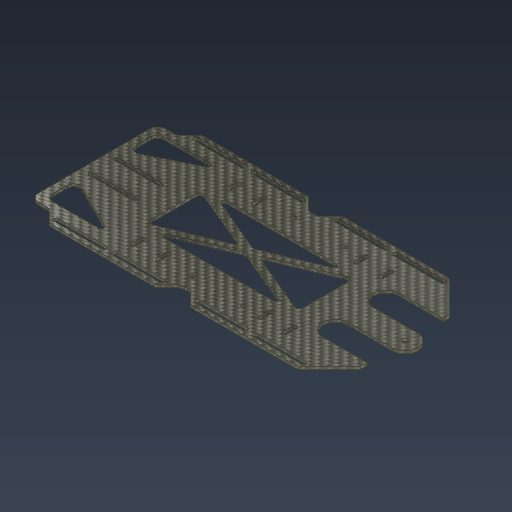
# Autodesk Inventor part: Battery_Tray
Saved by Autodesk Inventor 2024.1 (Build 281209000, 209)
## iProperties
Created: 2023-06-19
Part Number: Battery_Tray
Material: CFRP
Document SubType Name: Modeling
Designer: dzw04
Density: 1.43 g/cm^3
Appearance: Carbon Fiber 1
Mass: 54.159 g
Surface Area: 436.496 cm^2
Volume: 37.8734 cm^3
Author: dzw04
Autodesk Inventor part; units mm, degrees
ref_plane "YZ Plane" through (0, 0, 0) normal (1, 0, 0) x (0, 1, 0)
ref_plane "XZ Plane" through (0, 0, 0) normal (0, 1, 0) x (-1, 0, 0)
ref_plane "XY Plane" through (0, 0, 0) normal (0, 0, 1) x (1, 0, 0)
sketch "Sketch1" plane through (0, 0, 0) normal (0, 1, 0) x (-1, 0, 0)
  line L0 (-110, 36.5) -> (110, 36.5) construction
  line L1 (110, 36.5) -> (110, -36.5) construction
  line L2 (110, -36.5) -> (-110, -36.5) construction
  line L3 (-110, -36.5) -> (-110, 36.5) construction
  line L4 (-110, 36.5) -> (110, -36.5) construction
  line L5 (110, 36.5) -> (-110, -36.5) construction
  line L6 (-110, 29) -> (80, 29) construction
  line L7 (80, 29) -> (80, -29) construction
  line L8 (80, -29) -> (-110, -29) construction
  line L9 (-110, -29) -> (-110, 29) construction
  line L10 (-110, 29) -> (80, -29) construction
  line L11 (80, 29) -> (-110, -29) construction
  line L12 (-110, -29) -> (-110, -34) construction
  line L13 (-110, -34) -> (-60, -34) construction
  line L14 (-60, -34) -> (-50, -34) construction
  line L15 (-50, -34) -> (-70, -34) construction
  line L16 (-50, -34) -> (-50, -41.5) construction
  line L17 (-51.5, -34) -> (-51.5, -41.5)
  line L18 (-48.5, -41.5) -> (-48.5, -34)
  arc A0 (-48.5, -34) -> (-51.5, -34) centre (-50, -34) ccw
  arc A1 (-51.5, -41.5) -> (-48.5, -41.5) centre (-50, -41.5) ccw
  line L19 (-70, -34) -> (-70, -41.5) construction
  line L20 (-71.5, -34) -> (-71.5, -41.5)
  line L21 (-68.5, -41.5) -> (-68.5, -34)
  arc A2 (-68.5, -34) -> (-71.5, -34) centre (-70, -34) ccw
  arc A3 (-71.5, -41.5) -> (-68.5, -41.5) centre (-70, -41.5) ccw
  line L22 (122.5, 50) -> (-122.5, 50)
  line L23 (-122.5, 50) -> (-122.5, -50)
  line L24 (-122.5, -50) -> (122.5, -50)
  line L25 (122.5, -50) -> (122.5, 50)
  line L26 (122.5, 50) -> (-122.5, -50) construction
  line L27 (-122.5, 50) -> (122.5, -50) construction
  line L28 (122.5, 0) -> (-124.7912, 0) construction
  line L29 (-50, -34) -> (30, -34) construction
  line L30 (30, -34) -> (50, -34) construction
  line L31 (30, -34) -> (30, -41.5) construction
  line L32 (28.5, -34) -> (28.5, -41.5)
  line L33 (31.5, -41.5) -> (31.5, -34)
  arc A4 (31.5, -34) -> (28.5, -34) centre (30, -34) ccw
  arc A5 (28.5, -41.5) -> (31.5, -41.5) centre (30, -41.5) ccw
  line L34 (50, -34) -> (50, -41.5) construction
  line L35 (48.5, -34) -> (48.5, -41.5)
  line L36 (51.5, -41.5) -> (51.5, -34)
  arc A6 (51.5, -34) -> (48.5, -34) centre (50, -34) ccw
  arc A7 (48.5, -41.5) -> (51.5, -41.5) centre (50, -41.5) ccw
  line L37 (-110, 0) -> (80, 0) construction
  line L38 (80, 0) -> (80, -10) construction
  line L39 (80, 0) -> (80, 10) construction
  line L40 (80, -10) -> (115, -10) construction
  line L41 (80, -11.5) -> (115, -11.5)
  line L42 (115, -8.5) -> (80, -8.5)
  arc A8 (80, -8.5) -> (80, -11.5) centre (80, -10) ccw
  arc A9 (115, -11.5) -> (115, -8.5) centre (115, -10) ccw
  line L43 (80, 10) -> (115, 10) construction
  line L44 (80, 8.5) -> (115, 8.5)
  line L45 (115, 11.5) -> (80, 11.5)
  arc A10 (80, 11.5) -> (80, 8.5) centre (80, 10) ccw
  arc A11 (115, 8.5) -> (115, 11.5) centre (115, 10) ccw
  line L46 (-60, 34) -> (-50, 34) construction
  line L47 (-50, 34) -> (-70, 34) construction
  line L48 (-50, 34) -> (-50, 41.5) construction
  line L49 (-51.5, 34) -> (-51.5, 41.5)
  line L50 (-48.5, 41.5) -> (-48.5, 34)
  arc A12 (-51.5, 34) -> (-48.5, 34) centre (-50, 34) ccw
  arc A13 (-48.5, 41.5) -> (-51.5, 41.5) centre (-50, 41.5) ccw
  line L51 (-70, 34) -> (-70, 41.5) construction
  line L52 (-71.5, 34) -> (-71.5, 41.5)
  line L53 (-68.5, 41.5) -> (-68.5, 34)
  arc A14 (-71.5, 34) -> (-68.5, 34) centre (-70, 34) ccw
  arc A15 (-68.5, 41.5) -> (-71.5, 41.5) centre (-70, 41.5) ccw
  line L54 (-50, 34) -> (30, 34) construction
  line L55 (30, 34) -> (50, 34) construction
  line L56 (30, 34) -> (30, 41.5) construction
  line L57 (28.5, 34) -> (28.5, 41.5)
  line L58 (31.5, 41.5) -> (31.5, 34)
  arc A16 (28.5, 34) -> (31.5, 34) centre (30, 34) ccw
  arc A17 (31.5, 41.5) -> (28.5, 41.5) centre (30, 41.5) ccw
  line L59 (50, 34) -> (50, 41.5) construction
  line L60 (48.5, 34) -> (48.5, 41.5)
  line L61 (51.5, 41.5) -> (51.5, 34)
  arc A18 (48.5, 34) -> (51.5, 34) centre (50, 34) ccw
  arc A19 (51.5, 41.5) -> (48.5, 41.5) centre (50, 41.5) ccw
  circle A20 centre (-122.5, 0) radius 10
  point P0 (0, 0)
  point P1 (-15, 0)
  point P2 (-50, -37.75)
  point P3 (-70, -37.75)
  point P4 (30, -37.75)
  point P5 (50, -37.75)
  point P6 (97.5, -10)
  point P7 (97.5, 10)
  point P8 (-50, 37.75)
  point P9 (-70, 37.75)
  point P10 (30, 37.75)
  point P11 (50, 37.75)
  point P12 (-122.5, -10)
  point P13 (-122.5, 10)
  dimension "d0" = 220
  dimension "d1" = 73
  dimension "d2" = 190
  dimension "d3" = 58
  dimension "d4" = 5
  dimension "d5" = 50
  dimension "d6" = 10
  dimension "d7" = 20
  dimension "d8" = 7.5
  dimension "d9" = 3
  dimension "d10" = 7.5
  dimension "d11" = 3
  dimension "d12" = 245
  dimension "d13" = 100
  dimension "d16" = 80
  dimension "d17" = 20
  dimension "d18" = 7.5
  dimension "d19" = 3
  dimension "d20" = 7.5
  dimension "d21" = 3
  dimension "d22" = 10
  dimension "d23" = 10
  dimension "d24" = 35
  dimension "d25" = 3
  dimension "d26" = 35
  dimension "d27" = 3
  dimension "d52" = 20
  constraints: 144 end point, 40 point on circle, 29 symmetric about line, 24 tangent, 21 centre point, 17 midpoint, 14 parallel, 11 point on line, 8 perpendicular, 3 horizontal, 1 vertical, 8 other
  measures "d0" distance of L1.end L2.end
  measures "d1" distance of L0.end L1.end
  measures "d2" distance of L7.end L8.end
  measures "d3" distance of L6.end L7.end
  measures "d4" distance of L8.end L12.end
  measures "d5" distance of L12.end L13.end
  measures "d6" distance of L13.end L14.end
  measures "d7" distance of L14.end L15.end
  measures "d8" distance of L14.end L16.end
  measures "d9" diameter of A1
  measures "d10" distance of L15.end L19.end
  measures "d11" diameter of A3
  measures "d12" distance of L24.end L23.end
  measures "d13" distance of L23.end L22.end
  measures "d16" distance of L14.end L29.end
  measures "d17" distance of L29.end L30.end
  measures "d18" distance of L29.end L31.end
  measures "d19" diameter of A5
  measures "d20" distance of L30.end L34.end
  measures "d21" diameter of A7
  measures "d22" distance of L37.end L38.end
  measures "d23" distance of L37.end L39.end
  measures "d24" distance of L38.end L40.end
  measures "d25" diameter of A9
  measures "d26" distance of L39.end L43.end
  measures "d27" diameter of A11
  measures "d52" diameter of A20
extrude "Extrusion1" add sketch "Sketch1" along normal blind 2
sketch "Sketch2" plane through (0, 2, 0) normal (0, 1, 0) x (1, 0, 0)
  line L0 (0, 0) -> (55.5, 0) construction
  line L1 (55.5, 0) -> (55.5, -55) construction
  line L2 (55.5, -55) -> (51.5, -55) construction
  line L3 (51.5, -55) -> (14, -55) construction
  line L4 (51.5, -53.25) -> (14, -53.25)
  line L5 (14, -56.75) -> (51.5, -56.75)
  arc A0 (51.5, -56.75) -> (51.5, -53.25) centre (51.5, -55) ccw
  arc A1 (14, -53.25) -> (14, -56.75) centre (14, -55) ccw
  line L6 (14, -55) -> (28.5, -55) construction
  line L7 (28.5, -55) -> (13.5, -55) construction
  line L8 (0, 0) -> (0, -30) construction
  line L9 (55.5, -55) -> (59.5, -55) construction
  line L10 (59.5, -55) -> (97, -55) construction
  line L11 (59.5, -53.25) -> (97, -53.25)
  line L12 (97, -56.75) -> (59.5, -56.75)
  arc A2 (59.5, -53.25) -> (59.5, -56.75) centre (59.5, -55) ccw
  arc A3 (97, -56.75) -> (97, -53.25) centre (97, -55) ccw
  line L13 (97, -55) -> (82.5, -55) construction
  line L14 (82.5, -55) -> (97.5, -55) construction
  line L15 (82.5, -53.25) -> (97.5, -53.25)
  line L16 (97.5, -56.75) -> (82.5, -56.75)
  arc A4 (82.5, -53.25) -> (82.5, -56.75) centre (82.5, -55) ccw
  arc A5 (97.5, -56.75) -> (97.5, -53.25) centre (97.5, -55) ccw
  line L17 (-122.5, -50) -> (122.5, -50) projected
  line L18 (122.5, -50) -> (109.5711, -50)
  line L19 (107.5, -50) -> (107.5, -60) construction
  line L20 (107.5, -60) -> (97.5, -60) construction
  line L21 (98.9645, -58.5355) -> (106.0355, -51.4645)
  line L22 (95.4289, -60) -> (50.5, -60)
  arc A6 (95.4289, -60) -> (98.9645, -58.5355) centre (95.4289, -55) ccw
  arc A7 (109.5711, -50) -> (106.0355, -51.4645) centre (109.5711, -55) ccw
  line L23 (12.0355, -58.5355) -> (4.9645, -51.4645)
  line L24 (15.5711, -60) -> (50.5, -60)
  arc A8 (12.0355, -58.5355) -> (15.5711, -60) centre (15.5711, -55) ccw
  arc A9 (4.9645, -51.4645) -> (1.4289, -50) centre (1.4289, -55) ccw
  line L25 (-55.5, 0) -> (-55.5, -55) construction
  line L26 (-55.5, -55) -> (-51.5, -55) construction
  line L27 (-51.5, -55) -> (-14, -55) construction
  line L28 (-51.5, -53.25) -> (-14, -53.25)
  line L29 (-14, -56.75) -> (-51.5, -56.75)
  arc A10 (-51.5, -53.25) -> (-51.5, -56.75) centre (-51.5, -55) ccw
  arc A11 (-14, -56.75) -> (-14, -53.25) centre (-14, -55) ccw
  line L30 (-14, -55) -> (-28.5, -55) construction
  line L31 (-28.5, -55) -> (-13.5, -55) construction
  line L32 (-28.5, -53.25) -> (-13.5, -53.25)
  line L33 (-13.5, -56.75) -> (-28.5, -56.75)
  arc A12 (-28.5, -53.25) -> (-28.5, -56.75) centre (-28.5, -55) ccw
  arc A13 (-13.5, -56.75) -> (-13.5, -53.25) centre (-13.5, -55) ccw
  line L34 (-97, -56.75) -> (-59.5, -56.75)
  arc A14 (-59.5, -56.75) -> (-59.5, -53.25) centre (-59.5, -55) ccw
  arc A15 (-97, -53.25) -> (-97, -56.75) centre (-97, -55) ccw
  line L35 (-97, -55) -> (-82.5, -55) construction
  arc A16 (-82.5, -56.75) -> (-82.5, -53.25) centre (-82.5, -55) ccw
  line L36 (-97.5, -56.75) -> (-82.5, -56.75)
  arc A17 (-97.5, -53.25) -> (-97.5, -56.75) centre (-97.5, -55) ccw
  line L37 (-82.5, -55) -> (-97.5, -55) construction
  line L38 (-82.5, -53.25) -> (-97.5, -53.25)
  line L39 (-59.5, -55) -> (-97, -55) construction
  line L40 (-59.5, -53.25) -> (-97, -53.25)
  line L41 (-55.5, -55) -> (-59.5, -55) construction
  line L42 (122.5, -50) -> (-122.5, -50)
  line L43 (-122.5, -50) -> (-109.5711, -50)
  line L44 (-107.5, -50) -> (-107.5, -60) construction
  line L45 (-107.5, -60) -> (-97.5, -60) construction
  line L46 (-98.9645, -58.5355) -> (-106.0355, -51.4645)
  line L47 (-95.4289, -60) -> (-50.5, -60)
  arc A18 (-98.9645, -58.5355) -> (-95.4289, -60) centre (-95.4289, -55) ccw
  arc A19 (-106.0355, -51.4645) -> (-109.5711, -50) centre (-109.5711, -55) ccw
  line L48 (-15.5711, -60) -> (-50.5, -60)
  arc A20 (-15.5711, -60) -> (-12.0355, -58.5355) centre (-15.5711, -55) ccw
  line L49 (-12.0355, -58.5355) -> (-4.9645, -51.4645)
  arc A21 (-1.4289, -50) -> (-4.9645, -51.4645) centre (-1.4289, -55) ccw
  line L50 (55.5, 0) -> (55.5, 55) construction
  line L51 (55.5, 55) -> (51.5, 55) construction
  line L52 (51.5, 55) -> (14, 55) construction
  line L53 (51.5, 53.25) -> (14, 53.25)
  line L54 (14, 56.75) -> (51.5, 56.75)
  arc A22 (51.5, 53.25) -> (51.5, 56.75) centre (51.5, 55) ccw
  arc A23 (14, 56.75) -> (14, 53.25) centre (14, 55) ccw
  line L55 (14, 55) -> (28.5, 55) construction
  line L56 (28.5, 55) -> (13.5, 55) construction
  line L57 (28.5, 53.25) -> (13.5, 53.25)
  line L58 (13.5, 56.75) -> (28.5, 56.75)
  arc A24 (28.5, 53.25) -> (28.5, 56.75) centre (28.5, 55) ccw
  arc A25 (13.5, 56.75) -> (13.5, 53.25) centre (13.5, 55) ccw
  line L59 (97, 56.75) -> (59.5, 56.75)
  arc A26 (59.5, 56.75) -> (59.5, 53.25) centre (59.5, 55) ccw
  arc A27 (97, 53.25) -> (97, 56.75) centre (97, 55) ccw
  line L60 (97, 55) -> (82.5, 55) construction
  arc A28 (82.5, 56.75) -> (82.5, 53.25) centre (82.5, 55) ccw
  line L61 (97.5, 56.75) -> (82.5, 56.75)
  arc A29 (97.5, 53.25) -> (97.5, 56.75) centre (97.5, 55) ccw
  line L62 (82.5, 55) -> (97.5, 55) construction
  line L63 (82.5, 53.25) -> (97.5, 53.25)
  line L64 (59.5, 55) -> (97, 55) construction
  line L65 (59.5, 53.25) -> (97, 53.25)
  line L66 (55.5, 55) -> (59.5, 55) construction
  line L67 (-122.5, 50) -> (122.5, 50)
  line L68 (122.5, 50) -> (109.5711, 50)
  line L69 (107.5, 50) -> (107.5, 60) construction
  line L70 (107.5, 60) -> (97.5, 60) construction
  line L71 (98.9645, 58.5355) -> (106.0355, 51.4645)
  line L72 (95.4289, 60) -> (50.5, 60)
  arc A30 (98.9645, 58.5355) -> (95.4289, 60) centre (95.4289, 55) ccw
  arc A31 (106.0355, 51.4645) -> (109.5711, 50) centre (109.5711, 55) ccw
  line L73 (15.5711, 60) -> (50.5, 60)
  arc A32 (15.5711, 60) -> (12.0355, 58.5355) centre (15.5711, 55) ccw
  line L74 (12.0355, 58.5355) -> (4.9645, 51.4645)
  arc A33 (1.4289, 50) -> (4.9645, 51.4645) centre (1.4289, 55) ccw
  line L75 (-55.5, 55) -> (-51.5, 55) construction
  line L76 (-14, 55) -> (-28.5, 55) construction
  line L77 (122.5, 50) -> (-122.5, 50)
  line L78 (-15.5711, 60) -> (-50.5, 60)
  arc A34 (-14, 53.25) -> (-14, 56.75) centre (-14, 55) ccw
  line L79 (-51.5, 55) -> (-14, 55) construction
  line L80 (-14, 56.75) -> (-51.5, 56.75)
  arc A35 (-51.5, 56.75) -> (-51.5, 53.25) centre (-51.5, 55) ccw
  arc A36 (-59.5, 53.25) -> (-59.5, 56.75) centre (-59.5, 55) ccw
  line L81 (-51.5, 53.25) -> (-14, 53.25)
  arc A37 (-28.5, 56.75) -> (-28.5, 53.25) centre (-28.5, 55) ccw
  line L82 (-28.5, 53.25) -> (-13.5, 53.25)
  line L83 (-28.5, 55) -> (-13.5, 55) construction
  line L84 (-13.5, 56.75) -> (-28.5, 56.75)
  arc A38 (-13.5, 53.25) -> (-13.5, 56.75) centre (-13.5, 55) ccw
  arc A39 (-12.0355, 58.5355) -> (-15.5711, 60) centre (-15.5711, 55) ccw
  line L85 (-12.0355, 58.5355) -> (-4.9645, 51.4645)
  arc A40 (-4.9645, 51.4645) -> (-1.4289, 50) centre (-1.4289, 55) ccw
  line L86 (-55.5, 0) -> (-55.5, 55) construction
  line L87 (-59.5, 55) -> (-97, 55) construction
  arc A41 (-97, 56.75) -> (-97, 53.25) centre (-97, 55) ccw
  line L88 (-97, 55) -> (-82.5, 55) construction
  arc A42 (-82.5, 53.25) -> (-82.5, 56.75) centre (-82.5, 55) ccw
  line L89 (-82.5, 53.25) -> (-97.5, 53.25)
  line L90 (-82.5, 55) -> (-97.5, 55) construction
  line L91 (-97.5, 56.75) -> (-82.5, 56.75)
  arc A43 (-97.5, 56.75) -> (-97.5, 53.25) centre (-97.5, 55) ccw
  line L92 (-97, 56.75) -> (-59.5, 56.75)
  line L93 (-55.5, 55) -> (-59.5, 55) construction
  line L94 (-59.5, 53.25) -> (-97, 53.25)
  arc A44 (-95.4289, 60) -> (-98.9645, 58.5355) centre (-95.4289, 55) ccw
  line L95 (-98.9645, 58.5355) -> (-106.0355, 51.4645)
  line L96 (-107.5, 50) -> (-107.5, 60) construction
  line L97 (-107.5, 60) -> (-97.5, 60) construction
  arc A45 (-109.5711, 50) -> (-106.0355, 51.4645) centre (-109.5711, 55) ccw
  line L98 (-122.5, 50) -> (-109.5711, 50)
  line L99 (-95.4289, 60) -> (-50.5, 60)
  line L100 (122.5, 10) -> (122.5, 50) projected
  line L101 (122.5, 10) -> (87.5, 10)
  line L102 (122.5, -50) -> (122.5, -10) projected
  line L103 (122.5, -10) -> (87.5, -10)
  line L104 (87.5, 10) -> (87.5, 30) construction
  line L105 (87.5, -10) -> (87.5, -30) construction
  line L106 (87.5, 30) -> (122.5, 30)
  line L107 (87.5, -30) -> (122.5, -30)
  arc A46 (87.5, 30) -> (87.5, 10) centre (87.5, 20) ccw
  arc A47 (87.5, -10) -> (87.5, -30) centre (87.5, -20) ccw
  point P0 (32.75, -55)
  point P1 (21, -55)
  point P2 (78.25, -55)
  point P3 (90, -55)
  point P4 (-32.75, -55)
  point P5 (-21, -55)
  point P6 (-90, -55)
  point P7 (-78.25, -55)
  point P8 (32.75, 55)
  point P9 (21, 55)
  point P10 (90, 55)
  point P11 (78.25, 55)
  point P12 (-32.75, 55)
  point P13 (-21, 55)
  point P14 (-90, 55)
  point P15 (-78.25, 55)
  point P16 (1.4289, 50)
  point P17 (109.5711, 50)
  point P18 (-109.5711, 50)
  point P19 (-1.4289, 50)
  point P20 (-1.4289, -50)
  point P21 (-109.5711, -50)
  point P22 (109.5711, -50)
  point P23 (1.4289, -50)
  dimension "d28" = 55.5
  dimension "d29" = 55
  dimension "d30" = 4
  dimension "d31" = 37.5
  dimension "d32" = 3.5
  dimension "d36" = 30
  dimension "d37" = 15
  dimension "d38" = 10
  dimension "d39" = 10
  dimension "d40" = 5
  dimension "d53" = 35
  dimension "d54" = 35
  dimension "d55" = 20
  dimension "d56" = 20
  constraints: 241 end point, 147 symmetric about line, 96 point on circle, 48 centre point, 27 point on line, 8 tangent, 7 horizontal, 6 midpoint, 4 vertical, 2 perpendicular, 1 equal radius, 1 parallel, 36 other
  measures "d28" distance of L0.start L0.end
  measures "d29" distance of L0.end L1.end
  measures "d30" distance of L1.end L2.end
  measures "d31" distance of L2.end L3.end
  measures "d32" diameter of A1
  measures "d36" distance of L0.start L8.end
  measures "d37" distance of L17.end L19.start
  measures "d38" distance of L19.start L19.end
  measures "d39" distance of L19.end L20.end
  measures "d40" radius of A6
  measures "d53" distance of L100.start L101.end
  measures "d54" distance of L102.end L103.end
  measures "d55" distance of L101.end L104.end
  measures "d56" distance of L103.end L105.end
extrude "Extrusion2" add sketch "Sketch2" against normal blind 2 contours L17 A7 L21 A6 L22 L24 A8 L23 A9 | L17 A21 L49 A20 L48 L47 A18 L46 A19 | A45 L95 A44 L99 L78 A39 L85 A40 L67 | A33 L74 A32 L73 L72 A30 L71 A31 L67
sketch "Sketch3" plane through (0, 2, 0) normal (0, 1, 0) x (1, 0, 0)
  line L0 (98.9645, -58.5355) -> (106.0355, -51.4645) projected
  line L1 (106.0355, -51.4645) -> (137.8553, -19.6447)
  line L2 (106.0355, -51.4645) -> (151.0355, -51.4645) construction
  line L3 (106.0355, 51.4645) -> (137.8553, 19.6447)
  line L4 (106.0355, 51.4645) -> (151.0355, 51.4645) construction
  line L5 (106.0355, -51.4645) -> (127.5, -51.4645)
  line L6 (127.5, -51.4645) -> (127.5, -30)
  line L7 (127.5, -30) -> (106.0355, -30)
  line L8 (106.0355, -30) -> (106.0355, -51.4645)
  line L9 (106.0355, 51.4645) -> (127.5, 51.4645)
  line L10 (127.5, 51.4645) -> (127.5, 30)
  line L11 (127.5, 30) -> (106.0355, 30)
  line L12 (106.0355, 30) -> (106.0355, 51.4645)
  arc A0 (122.5, -10) -> (122.5, 10) centre (122.5, 0) ccw projected
  line L13 (122.5, 10) -> (87.5, 10)
  line L14 (87.5, 10) -> (87.5, 30) construction
  line L15 (87.5, 30) -> (122.5, 30)
  line L16 (122.5, 30) -> (122.5, 10)
  line L17 (122.5, -10) -> (87.5, -10)
  line L18 (87.5, -10) -> (87.5, -30) construction
  line L19 (87.5, -30) -> (122.5, -30)
  line L20 (122.5, -30) -> (122.5, -10)
  arc A1 (87.5, 30) -> (87.5, 10) centre (87.5, 20) ccw
  arc A2 (87.5, -10) -> (87.5, -30) centre (87.5, -20) ccw
  point P0 (0, 0)
  point P1 (122.5, 50)
  point P2 (106.0355, -30)
  point P3 (122.5, -30)
  point P4 (122.5, 30)
  point P5 (106.0355, 30)
  dimension "d43" = 45
  dimension "d44" = 45
  dimension "d45" = 45
  dimension "d46" = 45
  dimension "d57" = 35
  dimension "d58" = 20
  dimension "d59" = 35
  dimension "d60" = 20
  constraints: 40 end point, 8 parallel, 6 horizontal, 4 perpendicular, 4 point on circle, 2 centre point, 2 equal length, 2 midpoint, 2 point on line
  measures "d43" distance of L0.end L1.end
  measures "d44" angle of L2 L1
  measures "d45" distance of L3.start L3.end
  measures "d46" angle of L3 L4
  measures "d57" distance of L14.end L15.end
  measures "d58" distance of L13.end L14.end
  measures "d59" distance of L19.end L18.end
  measures "d60" distance of L18.end L17.end
extrude "Extrusion3" cut sketch "Sketch3" against normal through all contours L1 L6 L5 | L13 A1 L15 L11 L16 | L19 A2 L17 L20 L7 | L3 L9 L10
fillet "Fillet1" radius 6 2 edges at (-122.5, 1, -50) (-122.5, 1, 50)
sketch "Sketch5" plane through (0, 2, 0) normal (0, 1, 0) x (1, 0, 0)
  line L0 (0, 0) -> (15, 0) construction
  line L1 (35, -40) -> (-5, -40) construction
  line L2 (-5, -40) -> (-5, 40) construction
  line L3 (-5, 40) -> (35, 40) construction
  line L4 (35, 40) -> (35, -40) construction
  line L5 (35, -40) -> (-5, 40) construction
  line L6 (-5, -40) -> (35, 40) construction
  circle A0 centre (35, -40) radius 1.75
  circle A1 centre (35, 40) radius 1.75
  circle A2 centre (-5, 40) radius 1.75
  circle A3 centre (-5, -40) radius 1.75
  dimension "d61" = 15
  dimension "d62" = 40
  dimension "d63" = 80
  dimension "d64" = 3.5
  dimension "d65" = 3.5
  dimension "d66" = 3.5
  dimension "d67" = 3.5
  constraints: 14 end point, 4 centre point, 4 coincident, 2 horizontal, 2 midpoint, 2 parallel, 1 perpendicular
  measures "d61" distance of L0.start L0.end
  measures "d62" distance of L2.end L3.end
  measures "d63" distance of L1.end L2.end
  measures "d64" diameter of A0
  measures "d65" diameter of A1
  measures "d66" diameter of A2
  measures "d67" diameter of A3
extrude "Extrusion4" cut sketch "Sketch5" against normal through all
sketch "Sketch6" plane through (0, 2, 0) normal (0, 1, 0) x (1, 0, 0)
  arc A0 (122.5, -10) -> (122.5, 10) centre (122.5, 0) ccw projected
  circle A1 centre (122.5, 0) radius 12.5
  circle A2 centre (122.5, 0) radius 2.35
  point P0 (0, 0)
  dimension "d70" = 25
  dimension "d71" = 4.7
  constraints: 2 centre point, 2 coincident
  measures "d70" diameter of A1
  measures "d71" diameter of A2
extrude "Extrusion5" cut sketch "Sketch6" against normal through all contours A2
sketch "Sketch7" plane through (0, 2, 0) normal (0, 1, 0) x (1, 0, 0)
  line L0 (-43.5, -25) -> (43.5, -25)
  line L1 (60, -17.7917) -> (60, 17.7917)
  line L2 (43.5, 25) -> (-43.5, 25)
  line L3 (-60, 17.7917) -> (-60, -17.7917)
  line L4 (-60, -25) -> (60, 25) construction
  line L5 (60, -25) -> (-60, 25) construction
  line L6 (-55.8462, -20.5609) -> (-10.9308, -1.8462)
  line L7 (1.9231, 3.5096) -> (44.2692, 21.1538)
  line L8 (44.2692, -21.1538) -> (1.9231, -3.5096)
  line L9 (-10.9308, 1.8462) -> (-55.8462, 20.5609)
  line L10 (-44.2692, -21.1538) -> (-1.9231, -3.5096)
  line L11 (10.9308, 1.8462) -> (55.8462, 20.5609)
  line L12 (55.8462, -20.5609) -> (10.9308, -1.8462)
  line L13 (-1.9231, 3.5096) -> (-44.2692, 21.1538)
  arc A0 (-60, -17.7917) -> (-55.8462, -20.5609) centre (-57, -17.7917) ccw
  arc A1 (-55.8462, 20.5609) -> (-60, 17.7917) centre (-57, 17.7917) ccw
  arc A2 (60, 17.7917) -> (55.8462, 20.5609) centre (57, 17.7917) ccw
  arc A3 (55.8462, -20.5609) -> (60, -17.7917) centre (57, -17.7917) ccw
  arc A4 (43.5, -25) -> (44.2692, -21.1538) centre (43.5, -23) ccw
  arc A5 (44.2692, 21.1538) -> (43.5, 25) centre (43.5, 23) ccw
  arc A6 (-43.5, 25) -> (-44.2692, 21.1538) centre (-43.5, 23) ccw
  arc A7 (-44.2692, -21.1538) -> (-43.5, -25) centre (-43.5, -23) ccw
  arc A8 (10.9308, 1.8462) -> (10.9308, -1.8462) centre (11.7, 0) ccw
  arc A9 (-10.9308, -1.8462) -> (-10.9308, 1.8462) centre (-11.7, 0) ccw
  arc A10 (1.9231, -3.5096) -> (-1.9231, -3.5096) centre (0, -8.125) ccw
  arc A11 (-1.9231, 3.5096) -> (1.9231, 3.5096) centre (0, 8.125) ccw
  point P0 (0, 0)
  dimension "d76" = 120
  dimension "d77" = 50
  dimension "d82" = 3
  dimension "d83" = 2
  dimension "d84" = 5
  constraints: 28 end point, 24 point on circle, 24 tangent, 12 centre point, 10 parallel, 9 equal radius, 8 point on line, 2 midpoint, 1 horizontal, 1 perpendicular
  measures "d76" distance of L5.end L4.end
  measures "d77" distance of L4.end L5.start
  measures "d82" radius of A0
  measures "d83" radius of A4
  measures "d84" radius of A10
extrude "Extrusion6" cut sketch "Sketch7" against normal through all
sketch "Sketch8" plane through (0, 2, 0) normal (0, 1, 0) x (1, 0, 0)
  arc A0 (-116.5, 50) -> (-122.5, 44) centre (-116.5, 44) ccw projected
  line L0 (-111.5, 44) -> (-74.9721, 44)
  line L1 (-66.5, 44) -> (-66.5, 19) construction
  line L2 (-66.5, 19) -> (-116.5, 19) construction
  line L3 (-116.5, 27.0902) -> (-116.5, 39)
  arc A1 (-122.5, -44) -> (-116.5, -50) centre (-116.5, -44) ccw projected
  line L4 (-111.5, -44) -> (-74.9721, -44)
  line L5 (-66.5, -44) -> (-66.5, -19) construction
  line L6 (-66.5, -19) -> (-116.5, -19) construction
  line L7 (-116.5, -27.0902) -> (-116.5, -39)
  line L8 (-74.0777, -40.2111) -> (-109.2639, -22.618)
  line L9 (-109.2639, 22.618) -> (-74.0777, 40.2111)
  arc A2 (-116.5, -39) -> (-111.5, -44) centre (-111.5, -39) ccw
  arc A3 (-111.5, 44) -> (-116.5, 39) centre (-111.5, 39) ccw
  arc A4 (-109.2639, -22.618) -> (-116.5, -27.0902) centre (-111.5, -27.0902) ccw
  arc A5 (-116.5, 27.0902) -> (-109.2639, 22.618) centre (-111.5, 27.0902) ccw
  arc A6 (-74.9721, -44) -> (-74.0777, -40.2111) centre (-74.9721, -42) ccw
  arc A7 (-74.0777, 40.2111) -> (-74.9721, 44) centre (-74.9721, 42) ccw
  point P0 (0, 0)
  dimension "d87" = 50
  dimension "d88" = 25
  dimension "d89" = 50
  dimension "d90" = 25
  dimension "d91" = 5
  dimension "d92" = 5
  dimension "d93" = 2
  constraints: 20 end point, 12 point on circle, 12 point on line, 12 tangent, 6 centre point, 4 parallel, 3 equal radius, 2 horizontal, 2 perpendicular
  measures "d87" distance of L1.end L2.end
  measures "d88" distance of L1.start L1.end
  measures "d89" distance of L6.end L5.end
  measures "d90" distance of L5.end L5.start
  measures "d91" radius of A2
  measures "d92" radius of A4
  measures "d93" radius of A6
extrude "Extrusion7" cut sketch "Sketch8" against normal blind 3
equation "\"d14\" = ThicknessBatteryTray"
equation "\"d41\" = ThicknessBatteryTray"
equation "\"MountToMotorCenter\" = 0"
equation "\"ArmPosition\" = 5deg"
equation "\"BatteryWidth\" = 62"
equation "\"BatteryHeight\" = 76"
equation "\"ThicknessBodyOuterPlate\" = 2"
equation "\"ThicknessBodyCenterPlate\" = 2"
equation "\"ThicknessLegLoadpipePlate\" = 2"
equation "\"ThicknessBatteryTray\" = 2"
equation "\"ThicknessBatteryTopTray\" = 1"
equation "\"LandingGearStabilityBar\" = 525"
equation "\"StartAngleArm\" = 45deg"
equation "\"MotorMountCenter\" = 71.5"
body "Solid1"
